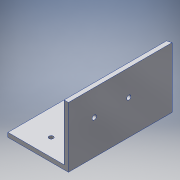
# Autodesk Inventor part: ring support right
Saved by Autodesk Inventor 2016 (Build 200138000, 138)
## iProperties
Created: 2015-02-06
Part Number: ring support right
Material: Aluminum 6061
Document SubType Name: Modeling
Designer: degan
Density: 2.7 g/cm^3
Appearance: Aluminum - Flat
Mass: 53.578 g
Surface Area: 135 cm^2
Volume: 19.8437 cm^3
Author: degan
Autodesk Inventor part; units mm, degrees
ref_plane "YZ Plane" through (0, 0, 0) normal (1, 0, 0) x (0, 1, 0)
ref_plane "XZ Plane" through (0, 0, 0) normal (0, 1, 0) x (-1, 0, 0)
sketch "Sketch1" plane through (0, 0, 0) normal (0, 0, 1) x (1, 0, 0)
  line L0 (0, 0) -> (0, 44.45)
  line L1 (0, 0) -> (-44.45, 0)
  line L2 (-3.175, 44.45) -> (-3.175, 3.175)
  line L3 (-3.175, 3.175) -> (-44.45, 3.175)
  line L4 (-3.175, 44.45) -> (0, 44.45)
  line L5 (-44.45, 3.175) -> (-44.45, 0)
  dimension "d0" = 44.45
  dimension "d1" = 44.45
  dimension "d2" = 3.175
  constraints: 12 end point, 3 perpendicular, 1 parallel, 1 vertical, 1 other
  measures "d0" distance of L0.start L0.end
  measures "d1" distance of L0.start L1.end
  measures "d2" distance between parallel lines of L0 L2
extrude "Extrusion1" add sketch "Sketch1" along normal blind 76.2
ref_plane "Work Plane1" through (0, 0, 0) normal (-0.2588, 0, -0.9659) x (0, 1, 0)
split "Split1" plane through (0, 0, 0) removes the side toward (-0.2588, 0, -0.9659)
sketch "Sketch2" plane through (-44.45, 3.175, 76.2) normal (0, 1, 0) x (1, 0, 0)
  line L0 (0, 0) -> (44.45, 0) projected
  circle A0 centre (19.05, 12.7) radius 2.0125
  circle A1 centre (19.05, 38.1) radius 1.8125
  line L1 (0, 64.2897) -> (0, 0) projected
  point P0 (44.45, 76.2)
  dimension "d6" = 12.7
  dimension "d7" = 25.4
  dimension "d28" = 19.05
  dimension "d29" = 19.05
  constraints: 2 centre point
  measures "d6" distance from line of L0 A0.centre
  measures "d7" distance of A0.centre A1.centre
  measures "d28" distance from line of A1.centre L1
  measures "d29" distance from line of L1 A0.centre
hole "Hole1" at (-25.4, 3.175, 38.1) at (-25.4, 3.175, 63.5) direction (0, -1, 0) diameter 3.175 end through all
sketch "Sketch3" plane through (-3.175, 3.175, 76.2) normal (-1, 0, 0) x (0, 0, 1)
  line L0 (0, -3.175) -> (0, 41.275)
  line L1 (-75.3493, 41.275) -> (-75.3493, 0)
  circle A0 centre (-19.05, 22.225) radius 1.7587
  circle A1 centre (-44.45, 22.225) radius 1.632
  line L2 (-75.3493, 41.275) -> (0, 41.275) projected
  point P0 (-76.2, -3.175)
  dimension "d15" = 19.05
  dimension "d16" = 25.4
  dimension "d26" = 19.05
  dimension "d27" = 19.05
  constraints: 4 end point, 2 centre point
  measures "d15" distance from line of A0.centre L0
  measures "d16" distance of A1.centre A0.centre
  measures "d26" distance from line of A1.centre L2
  measures "d27" distance from line of A0.centre L2
hole "Hole2" at (-3.175, 25.4, 31.75) at (-3.175, 25.4, 57.15) direction (1, 0, 0) diameter 3.175 end through all
body "Solid1"
